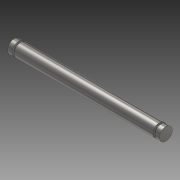
# Autodesk Inventor part: trolley_tendon_long_shaft
Saved by Autodesk Inventor 2017 SP1 (Build 210196100, 196)
## iProperties
Created: 2017-07-28
Part Number: trolley_tendon_long_shaft
Material: Stainless Steel
Document SubType Name: Modeling
Designer: JT
Density: 8 g/cm^3
Appearance: Semi-Polished
Author: JT
Autodesk Inventor part; units mm, degrees
ref_plane "YZ Plane" through (0, 0, 0) normal (1, 0, 0) x (0, 1, 0)
ref_plane "XZ Plane" through (0, 0, 0) normal (0, 1, 0) x (-1, 0, 0)
ref_plane "XY Plane" through (0, 0, 0) normal (0, 0, 1) x (1, 0, 0)
sketch "Sketch1" plane through (0, 0, 0) normal (0, 0, 1) x (1, 0, 0)
  line L0 (-11.8, 0) -> (11.8, 0)
  line L1 (-11.8, 0) -> (-11.8, 1)
  line L2 (-11.8, 1) -> (-11.1, 1)
  line L3 (-11.1, 1) -> (-11.1, 0.7)
  line L4 (-11.1, 0.7) -> (-10.8, 0.7)
  line L5 (-10.8, 0.7) -> (-10.8, 1)
  line L6 (-10.8, 1) -> (0, 1)
  line L7 (0, 0) -> (0, 5.9631) construction
  line L8 (11.8, 0) -> (11.8, 1)
  line L9 (11.8, 1) -> (11.1, 1)
  line L10 (11.1, 1) -> (11.1, 0.7)
  line L11 (11.1, 0.7) -> (10.8, 0.7)
  line L12 (10.8, 0.7) -> (10.8, 1)
  line L13 (10.8, 1) -> (0, 1)
  dimension "d0" = 23.6
  dimension "d1" = 0.3
  dimension "d2" = 21.6
  dimension "d3" = 2
  dimension "d4" = 1.4
  constraints: 28 end point, 6 symmetric about line, 4 perpendicular, 4 point on line, 2 vertical, 1 horizontal, 1 midpoint
  measures "d0" distance between parallel lines of L8 L1
  measures "d1" distance between parallel lines of L5 L3
  measures "d2" distance between parallel lines of L12 L5
  measures "d3" diameter of L6 L0
  measures "d4" diameter of L4 L0
revolve "Revolution1" add sketch "Sketch1" angle 360 about axis through (-11.8, 0, 0) along (1, 0, 0)
body "Solid1"
